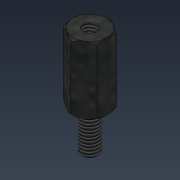
# Autodesk Inventor part: M2.5
Saved by Autodesk Inventor 2022.1 (Build 261234020, 234B)
## iProperties
Created: 2012-08-14
Part Number: M2.5
Material: Stahl
Document SubType Name: Modeling
Designer: rYan
Mass: 1.74537 g
Surface Area: 3.04272 cm^2
Volume: 0.22234 cm^3
Density: 7.85 g/cm^3
Appearance: Platte
Author: rYan
Autodesk Inventor part; units mm, degrees
ref_plane "YZ Plane" through (0, 0, 0) normal (1, 0, 0) x (0, 1, 0)
ref_plane "XZ Plane" through (0, 0, 0) normal (0, 1, 0) x (-1, 0, 0)
ref_plane "XY Plane" through (0, 0, 0) normal (0, 0, 1) x (1, 0, 0)
sketch "Skizze1" plane through (0, 0, 0) normal (0, 0, 1) x (1, 0, 0)
  line L0 (2.5, -1.4434) -> (0, -2.8868)
  line L1 (0, -2.8868) -> (-2.5, -1.4434)
  line L2 (-2.5, -1.4434) -> (-2.5, 1.4434)
  line L3 (-2.5, 1.4434) -> (0, 2.8868)
  line L4 (0, 2.8868) -> (2.5, 1.4434)
  line L5 (2.5, 1.4434) -> (2.5, -1.4434)
  line L6 (0, 4.4456) -> (0, -4.4456) projected
  point P0 (0, 0)
  point P1 (0, 0)
  dimension "SW" = 5
  constraints: 12 end point, 1 coincident, 1 parallel, 13 other
  measures "SW" distance between parallel lines of L2 L5
extrude "Extrusion1" add sketch "Skizze1" along normal mid plane 10
sketch "Skizze2" plane through (0, 0, 5) normal (0, 0, 1) x (1, 0, 0)
  point P0 (0, 0)
  point P1 (0, 0)
  constraints: 1 coincident
hole "Bohrung1" at (0, 0, 5) direction (0, 0, -1) diameter 2.013 depth 7 tip angle 118 thread size "M2.5x0.45" class "6H" standard "ISO Metric profile"
sketch "Skizze3" plane through (0, 0, -5) normal (0, 0, -1) x (-1, 0, 0)
  circle A0 centre (0, 0) radius 1.25
  dimension "GA_" = 2.5
  constraints: 1 centre point, 1 coincident
  measures "GA_" diameter of A0
extrude "Extrusion2" add sketch "Skizze3" along normal blind 6
thread "Gewinde1" size "M2.5x0.45" class "6g" standard "ANSI Metric M Profile" full length
chamfer "Fase1" distance 0.25 angle 45 1 edges at (1.25, 0, -11)
sketch "Skizze4" plane through (0, 0, 5) normal (0, 0, 1) x (1, 0, 0)
  line L0 (2.5, -1.4434) -> (2.5, 1.4434) projected
  circle A0 centre (0, 0) radius 2.5
  constraints: 1 centre point, 1 coincident, 1 tangent
sketch "Skizze5" plane through (0, 0, 0) normal (1, 0, 0) x (0, 1, 0)
  line L0 (-1.0065, 5) -> (1.0065, 5) projected
  line L1 (-2.8868, 5) -> (-1.4434, 5) projected
  line L2 (-1.4434, 5) -> (1.4434, 5) projected
  line L3 (1.4434, 5) -> (2.8868, 5) projected
  line L4 (2.8868, 5) -> (1.4434, 5) projected
  line L5 (1.4434, 5) -> (-1.4434, 5) projected
  line L6 (-1.4434, 5) -> (-2.8868, 5) projected
  line L7 (2.5, 5) -> (-2.5, 5) projected
  line L8 (2.8868, 5) -> (2.5, 5)
  line L9 (2.5, 5) -> (2.8868, 4.6132)
  line L10 (2.8868, 4.6132) -> (2.8868, 5)
  line L11 (0, 7) -> (0, -7) projected
  line L12 (1.25, -5) -> (-1.25, -5) projected
  line L13 (-1.4434, -5) -> (-2.8868, -5) projected
  line L14 (-2.8868, -5) -> (-1.4434, -5) projected
  line L15 (-1.4434, -5) -> (1.4434, -5) projected
  line L16 (1.4434, -5) -> (2.8868, -5) projected
  line L17 (2.8868, -5) -> (1.4434, -5) projected
  line L18 (1.4434, -5) -> (-1.4434, -5) projected
  line L19 (0, 5) -> (0, -5)
  point P0 (0, 0)
  dimension "d20" = 45
  constraints: 8 end point, 1 collinear, 1 midpoint, 1 perpendicular, 1 point on line, 2 other
  measures "d20" angle of L8 L9
revolve "Umdrehung1" cut sketch "Skizze5" angle 360 about axis through (0, 0, 5) along (0, 0, -1)
mirror "Spiegeln1" about plane through (0, 0, 0) normal (0, 0, 1) of "Umdrehung1"
